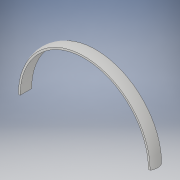
# Autodesk Inventor part: fender
Saved by Autodesk Inventor 2019 (Build 230136000, 136)
## iProperties
Created: 2019-10-03
Part Number: fender
Material: Generic
Document SubType Name: Modeling
Designer: Alex
Density: 1 g/cm^3
Appearance: Default
Author: Alex
Autodesk Inventor part; units mm, degrees
ref_plane "YZ Plane" through (0, 0, 0) normal (1, 0, 0) x (0, 1, 0)
ref_plane "XZ Plane" through (0, 0, 0) normal (0, 1, 0) x (-1, 0, 0)
ref_plane "XY Plane" through (0, 0, 0) normal (0, 0, 1) x (1, 0, 0)
sketch "Sketch1" plane through (0, 0, 0) normal (0, 1, 0) x (-1, 0, 0)
  line L0 (363, 32.5) -> (373, 32.5)
  line L1 (373, -32.5) -> (363, -32.5)
  arc A0 (373, -32.5) -> (373, 32.5) centre (319.5271, 0) ccw
  line L2 (363, 32.5) -> (363, -32.5)
  line L3 (0, 120.71) -> (0, -172.3479)
  point P0 (0, 0)
  dimension "d0" = 10
  dimension "d1" = 65
  dimension "d2" = 10
  dimension "d6" = 32.5
  dimension "d8" = 363
  constraints: 8 end point, 2 point on circle, 1 centre point, 1 horizontal, 1 parallel, 1 vertical
  measures "d0" distance of L0.start L0.end
  measures "d1" distance of L0.end L1.start
  measures "d2" distance of L1.start L1.end
  measures "d6" distance from line of point (0, 0) L0
  measures "d8" distance from line of point (0, 0) L2
revolve "Revolution1" add sketch "Sketch1" angle 180 about axis through (0, 0, 120.71) along (0, 0, -1)
body "Solid1"
